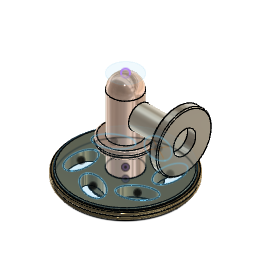
P6 (Autodesk Fusion 360 design; units mm, degrees)
Autodesk Fusion 360 part; units mm, degrees
sketch "Sketch1" plane through (0, 0, 0) normal (0, 0, 1) x (1, 0, 0)
  circle A0 centre (0, 0) radius 25
  dimension "d1" = 50
  constraint coincident A0.centre origin
  measures "d1" diameter of A0
extrude "Extrude1" add sketch "Sketch1" along normal blind 5 makes body 1
sketch "Sketch2" plane through (0, 0, 5) normal (0, 0, 1) x (-1, 0, 0)
  circle A0 centre (0, 0) radius 25
  ellipse E0 centre (0, -16) end of major axis (-6.9308, -12.4217) minor radius 4.35
  line L0 (6.9308, -19.5783) -> (-6.9308, -12.4217) construction
  line L1 (1.9956, -12.1348) -> (-1.9956, -19.8652) construction
  ellipse E1 centre (13.8564, -8) end of major axis (7.2921, -12.2131) minor radius 4.35
  ellipse E2 centre (13.8564, 8) end of major axis (14.2229, 0.2086) minor radius 4.35
  ellipse E3 centre (0, 16) end of major axis (6.9308, 12.4217) minor radius 4.35
  ellipse E4 centre (-13.8564, 8) end of major axis (-7.2921, 12.2131) minor radius 4.35
  ellipse E5 centre (-13.8564, -8) end of major axis (-14.2229, -0.2086) minor radius 4.35
  dimension "d5" = 16
  dimension "d15" = 360
  dimension "d16" = 7.8
  dimension "d17" = 8.7
  constraint coincident E0 L0.start
  constraint coincident E0 L0.end
  constraint coincident E0 L1.start
  constraint coincident E0 L1.end
  constraint vertical A0.centre E0.centre
  measures "d5" distance of A0.centre E0.centre
  measures "d16" distance of E0
sketch "Sketch3" plane through (0, 0, 5) normal (0, 0, 1) x (-1, 0, 0)
  circle A0 centre (0, 0) radius 25
  circle A1 centre (0, 0) radius 7
  dimension "d11" = 14
  constraint coincident A0.centre A1.centre
  measures "d11" diameter of A1
extrude "Extrude3" add sketch "Sketch3" along normal blind 40 separate body contours A1 makes body 2
extrude "Extrude4" cut sketch "Sketch2" against normal blind 10 contours E0 | E1 | E2 | E3 | E4 | E5 bodies 2 1
sketch "Sketch4" plane through (0, 0, 0) normal (0, 1, 0) x (1, 0, 0)
sketch "Sketch5" plane through (0, 0, 45) normal (0, 0, 1) x (-1, 0, 0)
  circle A0 centre (0, 0) radius 7
sketch "Sketch6" plane through (0, 0, 0) normal (0, 1, 0) x (1, 0, 0)
fillet "Fillet1" radius 7 1 faces at (-1.11, 1.8763, 45) on bodies 2
sketch "Sketch7" plane through (0, 0, 0) normal (0, 1, 0) x (1, 0, 0)
sketch "Sketch8" plane through (0, 0, 0) normal (1, 0, 0) x (0, 1, 0)
  circle A0 centre (0, 30) radius 5.5
  dimension "d30" = 30
  dimension "d31" = 11
  constraint vertical origin A0.centre
  measures "d30" distance of origin A0.centre
  measures "d31" diameter of A0
extrude "Extrude5" add sketch "Sketch8" along normal blind 18 from surface at 7 separate body makes body 3
sketch "Sketch9" plane through (25, 0, 0) normal (1, 0, 0) x (0, 1, 0)
  circle A0 centre (0, 30) radius 5.5
  circle A1 centre (0, 30) radius 13.5
  dimension "d35" = 27
  constraint concentric A0 A1
  measures "d35" diameter of A1
extrude "Extrude6" add sketch "Sketch9" along normal blind 4 separate body makes body 4
sketch "Sketch10" plane through (0, 0, 0) normal (1, 0, 0) x (0, 1, 0)
  line L0 (7, 5) -> (7, 19)
  line L1 (7, 19) -> (10, 19)
  arc A0 (10.8666, 17.501) -> (10, 19) centre (10, 18) ccw
  arc A1 (10.8666, 17.501) -> (10.8249, 16.5837) centre (11.7332, 17.002) ccw
  arc A2 (9.9166, 15.1654) -> (10.8249, 16.5837) centre (9.9166, 16.1654) ccw
  line L2 (9.9166, 15.1654) -> (7, 15.1654)
  point P0 (7, 15.1654)
  dimension "d38" = 14
  dimension "d39" = 3
  dimension "d40" = 1
  dimension "d41" = 1
  dimension "d42" = 1
  constraint vertical L0
  constraint tangent L1 A0
  constraint tangent A0 A1
  constraint tangent A1 A2
  constraint coincident L0 P0
  constraint horizontal L1
  constraint horizontal L2
  constraint tangent A2 L2
  constraint coincident L2 P0
  measures "d38" distance of L0.start L0.end
  measures "d39" distance of L0.end L1.end
  measures "d40" radius of A0
  measures "d41" radius of A1
  measures "d42" radius of A2
revolve "Revolve1" add sketch "Sketch10" angle 360 about axis through (0, 0, 5) along (0, 0, -1) bodies 2
sketch "Sketch11" plane through (0, 0, 0) normal (0, 1, 0) x (1, 0, 0)
  line L0 (25, 0) -> (25, -1)
  line L1 (25, -1) -> (25, -4)
  line L2 (25, -1) -> (26, -1)
  arc A0 (26, -2.2) -> (26, -1) centre (26, -1.6) ccw
  line L3 (26, -2.2) -> (26, -2.8)
  line L4 (25, -4) -> (26, -4)
  arc A1 (26, -4) -> (26, -2.8) centre (26, -3.4) ccw
  dimension "d44" = 1
  dimension "d45" = 3
  dimension "d46" = 1
  dimension "d47" = 0.6
  dimension "d48" = 0.6
  dimension "d49" = 1
  constraint vertical L0
  constraint parallel L0 L1
  constraint perpendicular L0 L2
  constraint tangent L2 A0
  constraint perpendicular L2 L3
  constraint perpendicular L1 L4
  constraint tangent L4 A1
  constraint horizontal L0.start origin
  constraint equal A0 A1
  measures "d44" distance of L0.start L0.end
  measures "d45" distance of L0.end L1.end
  measures "d46" distance of L0.end L2.end
  measures "d47" radius of A0
  measures "d48" distance of A0.start L3.end
  measures "d49" distance of L1.end L4.end
revolve "Revolve2" add sketch "Sketch11" angle 360 about axis through (0, 0, 0) along (0, 0, -1) bodies 1
fillet "Fillet2" radius 0.5 2 edges at (29, -12.5864, 25.1182) (25, -12.5864, 25.1182) on bodies 4
chamfer "Chamfer1" distance 0.5 angle 45 2 edges at (-23.3082, -9.0404, 0) (-23.3082, -9.0404, 5) on bodies 1
sketch "Sketch12" plane through (0, 0, 0) normal (0, 0, 1) x (1, 0, 0)
  circle A0 centre (0, 0) radius 13.5
  dimension "d54" = 27
  constraint coincident A0.centre origin
  measures "d54" diameter of A0
extrude "Extrude7" add sketch "Sketch12" against normal blind 0.5 bodies 1
